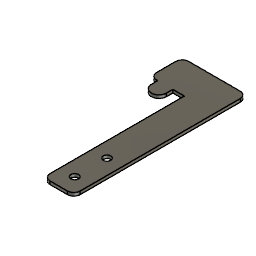
_Shelf Hangermount.b6095dcd-4930-469f-bd4d-1a79c03e5501 (Autodesk Fusion 360 design; units mm, degrees)
Autodesk Fusion 360 part; units mm, degrees
note: some values were not read from the file. Set by a fixed rule: which sketch regions a step uses.
sketch "Sketch1" plane through (0, 0, 0) normal (0, 0, 1) x (1, 0, 0) in component "Component"
  line L0 (0, 5) -> (0, 20.4)
  line L1 (5, 25.4) -> (45.8, 25.4)
  line L2 (5, 0) -> (6, 0)
  line L3 (6, 0) -> (18, 0) construction
  line L4 (12, 0) -> (12, -5) construction
  line L5 (6, 0) -> (6, -5)
  line L6 (18, 0) -> (18, -5)
  arc A0 (6, -5) -> (18, -5) centre (12, -5) ccw
  line L7 (18, 0) -> (27, 0)
  line L8 (27, 0) -> (27, -60)
  line L9 (50.8, 20.4) -> (50.8, -60)
  line L10 (27, -60) -> (50.8, -60) construction
  line L11 (50.8, -60) -> (50.8, -105.8)
  line L12 (45.8, -110.8) -> (32, -110.8)
  line L13 (27, -105.8) -> (27, -60)
  line L14 (50.8, -60) -> (27, -85.4) construction
  line L15 (50.8, -110.8) -> (27, -85.4) construction
  circle A1 centre (38.9, -72.7) radius 3
  circle A2 centre (38.9, -98.1) radius 3
  arc A3 (5, 25.4) -> (0, 20.4) centre (5, 20.4) ccw
  arc A4 (50.8, 20.4) -> (45.8, 25.4) centre (45.8, 20.4) ccw
  arc A5 (45.8, -110.8) -> (50.8, -105.8) centre (45.8, -105.8) ccw
  arc A6 (27, -105.8) -> (32, -110.8) centre (32, -105.8) ccw
  arc A7 (0, 5) -> (5, 0) centre (5, 5) ccw
  point P0 (0, 25.4)
  point P1 (50.8, 25.4)
  point P2 (27, -110.8)
  dimension "d2" = 50.8
  dimension "d3" = 25.4
  dimension "d4" = 6
  dimension "d6" = 5
  dimension "d7" = 60
  dimension "d9" = 50.8
  dimension "d10" = 6
  dimension "d14" = 6
  dimension "d15" = 5
  constraint vertical L0
  constraint perpendicular L0 L1
  constraint perpendicular L0 L2
  constraint parallel L2 L3
  constraint midpoint L3 L4.start
  constraint perpendicular L3 L4
  constraint coincident L4.end A0.centre
  constraint tangent L5 A0
  constraint perpendicular L3 L5
  constraint tangent L6 A0
  constraint perpendicular L6 L7
  constraint perpendicular L7 L8
  constraint perpendicular L1 L9
  constraint horizontal L10
  constraint vertical L11
  constraint horizontal L12
  constraint vertical L13
  constraint midpoint L14 A1.centre
  constraint midpoint L15 A2.centre
  constraint equal A1 A2
  constraint coincident P0 L0
  constraint coincident P0 L1
  constraint tangent L0 A3
  constraint tangent L1 A3
  constraint coincident P1 L1
  constraint coincident P1 L9
  constraint tangent L1 A4
  constraint tangent L9 A4
  constraint equal A3 A4
  constraint coincident L15.start L12
  constraint coincident L15.start L11
  constraint tangent L12 A5
  constraint tangent L11 A5
  constraint equal A3 A5
  constraint coincident L13 L14.end
  constraint coincident P2 L13
  constraint coincident P2 L12
  constraint tangent L13 A6
  constraint tangent L12 A6
  constraint equal A3 A6
  constraint coincident origin L2
  constraint coincident origin L0
  constraint tangent L2 A7
  constraint tangent L0 A7
  constraint equal A3 A7
  measures "d2" distance of P0 P1
  measures "d3" distance of origin P0
  measures "d4" distance of origin L2.end
  measures "d6" distance of L4.start L4.end
  measures "d7" distance of L7.end L8.end
  measures "d9" distance of L8.end P2
  measures "d10" diameter of A1
  measures "d14" radius of A0
  measures "d15" radius of A3
extrude "BaseFlange1" add sketch "Sketch1" along normal blind 2.5 in component "Component"
component "Component" placed x (1, 0, 0) y (0, 1, 0) z (0, 0, 1) at (0, 0, 0)
